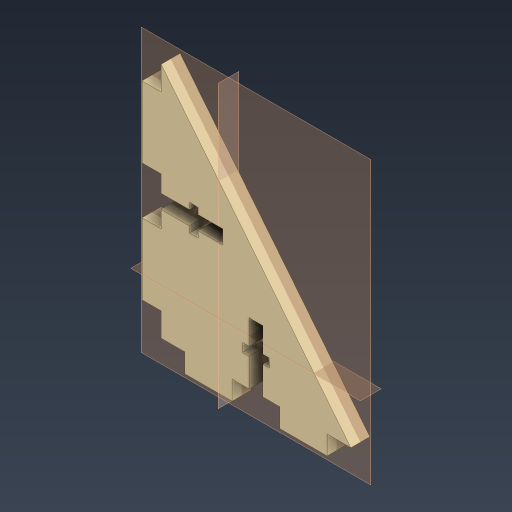
# Autodesk Inventor part: Рёбра_жёсткости
Saved by Autodesk Inventor 2023.2 (Build 272271030, 271C)
## iProperties
Created: 2025-12-29
Part Number: Рёбра_жёсткости
Material: Типовые
Document SubType Name: Modeling
Designer: Олег Коноваленко
Density: 1 g/cm^3
Appearance: Пшеничный
Author: Олег Коноваленко
Autodesk Inventor part; units mm, degrees
sketch "Эскиз1" plane through (0, 0, 0) normal (0, 0, 1) x (1, 0, 0)
  line L0 (-12.1951, 40.2439) -> (-12.1951, -9.7561)
  line L1 (-12.1951, -9.7561) -> (27.8049, -9.7561)
  line L2 (27.8049, -9.7561) -> (-12.1951, 40.2439)
  line L3 (-12.1951, -9.7561) -> (12.1951, 9.7561) construction
  line L4 (-7.1951, -9.7561) -> (2.8049, -9.7561)
  line L5 (2.8049, -9.7561) -> (2.8049, -13.7561)
  line L6 (2.8049, -13.7561) -> (-7.1951, -13.7561)
  line L7 (-7.1951, -13.7561) -> (-7.1951, -9.7561)
  line L8 (12.8049, -9.7561) -> (22.8049, -9.7561)
  line L9 (22.8049, -9.7561) -> (22.8049, -13.7561)
  line L10 (22.8049, -13.7561) -> (12.8049, -13.7561)
  line L11 (12.8049, -13.7561) -> (12.8049, -9.7561)
  line L12 (-12.1951, 35.2439) -> (-16.1951, 35.2439)
  line L13 (-16.1951, 35.2439) -> (-16.1951, 20.2439)
  line L14 (-16.1951, 20.2439) -> (-12.1951, 20.2439)
  line L15 (-12.1951, 20.2439) -> (-12.1951, 35.2439)
  line L16 (-12.1951, -4.7561) -> (-16.1951, -4.7561)
  line L17 (-16.1951, -4.7561) -> (-16.1951, 10.2439)
  line L18 (-16.1951, 10.2439) -> (-12.1951, 10.2439)
  line L19 (-12.1951, 10.2439) -> (-12.1951, -4.7561)
  point P0 (0, 0)
  point P1 (0, 0)
  point P2 (2.8049, -9.7561)
  dimension "d0" = 40
  dimension "d1" = 50
  dimension "d2" = 15
  dimension "d3" = 5
  dimension "d4" = 4
  dimension "d5" = 5
  dimension "d6" = 5
  dimension "d7" = 10
  dimension "d8" = 5
  constraints: 40 end point, 8 parallel, 6 perpendicular, 5 equal length, 5 point on line, 4 horizontal, 1 coincident, 1 midpoint, 1 vertical
  measures "d0" distance of L0.end L1.end
  measures "d1" distance of L0.start L0.end
  measures "d2" distance of L12.end L13.end
  measures "d3" distance from line of L0.start L12
  measures "d4" distance of L13.end L14.end
  measures "d5" distance from line of L0.end L16
  measures "d6" distance from line of L0.end L7
  measures "d7" distance of L5.end L6.end
  measures "d8" distance from line of L1.end L9
extrude "Выдавливание1" add sketch "Эскиз1" along normal mid plane 4
sketch "Эскиз2" plane through (0, 0, 2) normal (0, 0, 1) x (1, 0, 0)
  line L0 (-12.1951, 20.2439) -> (-12.1951, 10.2439) projected
  line L1 (-12.1951, 16.6939) -> (0.8049, 16.6939)
  line L2 (0.8049, 16.6939) -> (0.8049, 13.7939)
  line L3 (0.8049, 13.7939) -> (-12.1951, 13.7939)
  line L4 (-12.1951, 13.7939) -> (-12.1951, 16.6939)
  line L5 (2.8049, -9.7561) -> (12.8049, -9.7561) projected
  line L6 (6.3549, -9.7561) -> (9.2549, -9.7561)
  line L7 (9.2549, -9.7561) -> (9.2549, 3.2439)
  line L8 (9.2549, 3.2439) -> (6.3549, 3.2439)
  line L9 (6.3549, 3.2439) -> (6.3549, -9.7561)
  line L10 (-6.1951, 18.0439) -> (-4.3951, 18.0439)
  line L11 (-4.3951, 18.0439) -> (-4.3951, 12.4439)
  line L12 (-4.3951, 12.4439) -> (-6.1951, 12.4439)
  line L13 (-6.1951, 12.4439) -> (-6.1951, 18.0439)
  line L14 (5.0049, -1.9561) -> (10.6049, -1.9561)
  line L15 (10.6049, -1.9561) -> (10.6049, -3.7561)
  line L16 (10.6049, -3.7561) -> (5.0049, -3.7561)
  line L17 (5.0049, -3.7561) -> (5.0049, -1.9561)
  line L18 (-12.1951, 15.2439) -> (0.8049, 15.2439) construction
  line L19 (7.8049, 3.2439) -> (7.8049, -9.7561) construction
  point P0 (0, 0)
  point P1 (-4.3951, 15.2439)
  point P2 (7.8049, -1.9561)
  point P3 (-6.1951, 16.6939)
  point P4 (-6.1951, 13.7939)
  point P5 (-4.3951, 13.7939)
  point P6 (-4.3951, 16.6939)
  point P7 (6.3549, -3.7561)
  point P8 (9.2549, -3.7561)
  point P9 (9.2549, -1.9561)
  point P10 (6.3549, -1.9561)
  dimension "d11" = 2.9
  dimension "d12" = 13
  dimension "d13" = 1.8
  dimension "d14" = 5.6
  dimension "d15" = 6
  dimension "d16" = 6
  constraints: 36 end point, 8 midpoint, 8 parallel, 8 perpendicular, 4 horizontal, 4 point on line, 1 vertical
  measures "d11" distance of L1.end L2.end
  measures "d12" distance of L2.end L3.end
  measures "d13" distance of L10.start L10.end
  measures "d14" distance of L10.end L11.end
  measures "d15" distance between parallel lines of L0 L13
  measures "d16" distance between parallel lines of L5 L16
extrude "Выдавливание2" cut sketch "Эскиз2" against normal up to next
